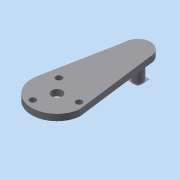
# Autodesk Inventor part: bras_codeur
Saved by Autodesk Inventor 2016 (Build 200138000, 138)
## iProperties
Created: 2017-01-03
Part Number: bras_codeur
Material: Generic
Document SubType Name: Modeling
Designer: Aegir
Density: 1 g/cm^3
Appearance: Default
Author: Aegir
Autodesk Inventor part; units mm, degrees
ref_plane "YZ Plane" through (0, 0, 0) normal (1, 0, 0) x (0, 1, 0)
ref_plane "XZ Plane" through (0, 0, 0) normal (0, 1, 0) x (-1, 0, 0)
sketch "Esquisse1" plane through (0, 0, 0) normal (0, 0, 1) x (1, 0, 0)
  circle A0 centre (-3.5, 0) radius 2.5 projected
  circle A1 centre (-3.5, 0) radius 2.5
  point P0 (0, 0)
  constraints: 1 centre point, 1 coincident, 1 concentric
ref_plane "Plan de construction1" through (-13, -9.5, -10) normal (0, 0, -1) x (0, 1, 0)
extrude "Extrusion1" add sketch "Esquisse1" against normal up to surface (10 mm away)
ref_plane "Plan de construction2" through (-3.5, 0, -9.5) normal (0, 0, -1) x (-1, 0, 0)
sketch "Esquisse2" plane through (-3.5, 0, -9.5) normal (0, 0, -1) x (-1, 0, 0)
  circle A0 centre (0, 0) radius 2.5
  circle A1 centre (0, 0) radius 2.2333
  point P0 (-3.5, 0)
  constraints: 2 centre point, 1 coincident
extrude "Extrusion2" cut sketch "Esquisse2" along normal mid plane 0.5
sketch "Esquisxse8" plane through (-3.5, 0, 0) normal (0, 0, 1) x (1, 0, 0)
  circle A0 centre (-1.0139, -37.4629) radius 12 projected
  circle A1 centre (-6.8791, -30.6366) radius 1.5 projected
  circle A2 centre (-3.9931, -45.9556) radius 1.5 projected
  circle A3 centre (7.8305, -35.7967) radius 1.5 projected
  circle A4 centre (0, 0) radius 2.5 projected
  arc A5 (6, 0) -> (-6, 0) centre (0, 0) ccw
  arc A6 (-12.7687, -35.0496) -> (10.3163, -33.5099) centre (-1.0139, -37.4629) ccw
  circle A7 centre (-3.9931, -45.9556) radius 1.5
  circle A8 centre (-6.8791, -30.6366) radius 1.5
  circle A9 centre (7.8305, -35.7967) radius 1.5
  line L0 (10.9482, -38.4158) -> (6, 0)
  line L1 (-6, 0) -> (-12.8221, -35.3258)
  point P0 (3.5, 0)
  dimension "d15" = 12
  constraints: 8 point on circle, 5 centre point, 5 coincident, 4 concentric, 4 end point, 2 point on line
  measures "d15" diameter of A5
extrude "Extrusion6" add sketch "Esquisxse8" along normal blind 3 contours L0 A0 | A0 L1 A5 L0 picked at (-1.038, -37.5266)
sketch "Esquisse9" plane through (-3.5, 0, 3) normal (0, 0, 1) x (1, 0, 0)
  circle A0 centre (0, 0) radius 2.5 projected
  circle A1 centre (0, 0) radius 2.5
  point P0 (3.5, 0)
  constraints: 1 centre point, 1 coincident, 1 concentric
extrude "Extrusion7" add sketch "Esquisse9" against normal blind 10
sketch "Esquisse11" plane through (-3.5, 0, 3) normal (0, 0, 1) x (1, 0, 0)
  circle A0 centre (-1.0139, -37.4629) radius 2.5
  point P0 (3.5, 0)
  constraints: 1 centre point, 2 other
extrude "Extrusion8" cut sketch "Esquisse11" against normal blind 10
